Y Pully Bonding Plate (Autodesk Fusion 360 design; units mm, degrees)
Autodesk Fusion 360 part; units mm, degrees
sketch "Sketch1" plane through (0, 0, 0) normal (0, 0, 1) x (1, 0, 0)
  line L0 (0, 0) -> (35, 0)
  line L1 (35, 0) -> (35, 16)
  line L2 (35, 16) -> (0, 16)
  line L3 (0, 16) -> (0, 0)
  dimension "d1" = 35
  dimension "d2" = 16
  constraint horizontal L0
  constraint vertical L1
  constraint horizontal L2
  constraint vertical L3
  constraint coincident L0.start L3.end
  measures "d1" distance of L0.start L0.end
  measures "d2" distance of L0.start L2.end
extrude "Extrude1" add sketch "Sketch1" along normal blind 2
sketch "Sketch2" plane through (0, 0, 2) normal (0, 0, 1) x (-1, 0, 0)
  line L0 (0, -16) -> (0, 0)
  line L1 (0, 0) -> (-35, 0)
  line L2 (-35, 0) -> (-35, -16)
  line L3 (-35, -16) -> (0, -16)
  circle A0 centre (-5, -8) radius 2.5
  circle A1 centre (-30, -8) radius 2.5
  dimension "d5" = 5
  dimension "d6" = 5
  dimension "d7" = 5
  measures "d5" diameter of A0
  measures "d6" distance of L0 A0.centre
  measures "d7" diameter of A1
extrude "Extrude2" cut sketch "Sketch2" against normal blind 6 contours A0 | A1
sketch "Sketch3" plane through (0, 0, 2) normal (0, 0, 1) x (-1, 0, 0)
  circle A0 centre (-30, -8) radius 2.5
  circle A1 centre (-5, -8) radius 2.5
  line L0 (0, -16) -> (0, 0)
  line L1 (0, 0) -> (-35, 0)
  line L2 (-35, 0) -> (-35, -16)
  line L3 (-35, -16) -> (0, -16)
  line L4 (-12, -6) -> (-24, -6) construction
  line L5 (-24, -6) -> (-24, -9) construction
  line L6 (-24, -9) -> (-12, -9) construction
  line L7 (-12, -9) -> (-12, -6) construction
  dimension "d10" = 8
  text T0 "lol" font "Arial" height 8 align left top in box 12 x 3 at (-12, -6) x (-1, 0) y (0, -1) spacing 1
extrude "Extrude3" add sketch "Sketch3" along normal blind 0.5 text T0
